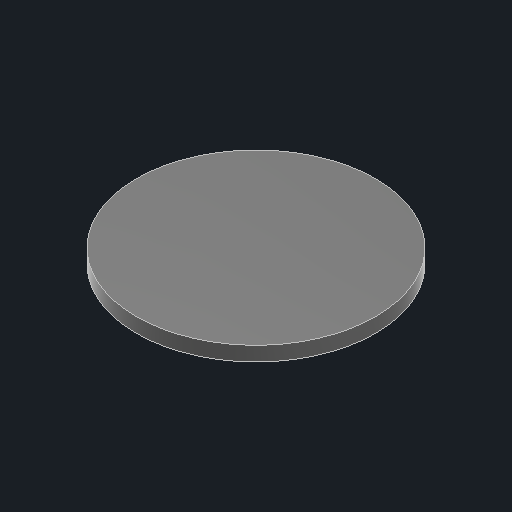
# Autodesk Inventor part: Foam Pad
Saved by Autodesk Inventor 2027.1 (Build 311270010, 270A)
## iProperties
Created: 2025-09-17
Material: Polystyrene
Document SubType Name: Modeling
Designer: SD
Density: 1.021 g/cm^3
Appearance: Smooth - Black
Mass: 0.848401 g
Surface Area: 9.75465 cm^2
Volume: 0.830951 cm^3
Project: Automatic Tea Steeping mechanism
Part Number: Foam Pad
BOM-Mass: 0.00085
BOM-Area: 0.001
Procurement: Buy
Build Stage: 3
Preferred Material: Manufacturer Specification
Author: SD
Title: Foam Pad
Autodesk Inventor part; units mm, degrees
ref_plane "YZ Plane" through (0, 0, 0) normal (1, 0, 0) x (0, 1, 0)
ref_plane "XZ Plane" through (0, 0, 0) normal (0, 1, 0) x (-1, 0, 0)
ref_plane "XY Plane" through (0, 0, 0) normal (0, 0, 1) x (1, 0, 0)
sketch "Sketch1" plane through (0, 0, 0) normal (0, 1, 0) x (-1, 0, 0)
  circle A0 centre (0, 0) radius 16.5
  dimension "d0" = 33
  constraints: 1 centre point, 1 coincident
  measures "d0" diameter of A0
extrude "Extrusion1" add sketch "Sketch1" along normal mid plane 2
body "Solid1"
